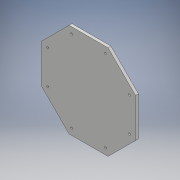
# Autodesk Inventor part: meteostanica radiation shield spodny kryt
Saved by Autodesk Inventor 2017 (Build 210142000, 142)
## iProperties
Created: 2017-02-23
Part Number: meteostanica radiation shield spodny kryt
Material: Generic
Document SubType Name: Modeling
Designer: Luc3as
Density: 1 g/cm^3
Appearance: Default
Author: Luc3as
Autodesk Inventor part; units mm, degrees
ref_plane "YZ Plane" through (0, 0, 0) normal (1, 0, 0) x (0, 1, 0)
ref_plane "XZ Plane" through (0, 0, 0) normal (0, 1, 0) x (-1, 0, 0)
ref_plane "XY Plane" through (0, 0, 0) normal (0, 0, 1) x (1, 0, 0)
ref_plane "Work Plane13" through (0, 0, 0) normal (0, -1, 0) x (1, 0, 0)
sketch "Sketch13" plane through (0, 0, 0) normal (0, -1, 0) x (1, 0, 0)
  circle A0 centre (-71.6992, -29.6988) radius 0.75 projected
  circle A1 centre (29.6988, -71.6992) radius 0.75 projected
  circle A2 centre (71.6992, 29.6988) radius 0.75 projected
  circle A3 centre (29.6988, 71.6992) radius 0.75 projected
  circle A4 centre (-29.6988, 71.6992) radius 0.75 projected
  circle A5 centre (71.6992, -29.6988) radius 0.75 projected
  circle A6 centre (-29.6988, -71.6992) radius 0.75 projected
  circle A7 centre (-71.6992, 29.6988) radius 0.75 projected
  line L0 (-82.6875, -34.2503) -> (-34.2503, -82.6875) projected
  line L1 (-34.2503, -82.6875) -> (34.2503, -82.6875) projected
  line L2 (34.2503, -82.6875) -> (82.6875, -34.2503) projected
  line L3 (82.6875, -34.2503) -> (82.6875, 34.2503) projected
  line L4 (82.6875, 34.2503) -> (34.2503, 82.6875) projected
  line L5 (34.2503, 82.6875) -> (-34.2503, 82.6875) projected
  line L6 (-34.2503, 82.6875) -> (-82.6875, 34.2503) projected
  line L7 (-82.6875, 34.2503) -> (-82.6875, -34.2503) projected
  arc A8 (-33.3536, 70.0737) -> (-25.965, 73.1342) centre (-29.6988, 71.6992) ccw projected
  arc A9 (25.965, 73.1342) -> (-25.965, 73.1342) centre (0, 0) ccw projected
  arc A10 (25.965, 73.1342) -> (33.3536, 70.0737) centre (29.6988, 71.6992) ccw projected
  arc A11 (70.0737, 33.3536) -> (33.3536, 70.0737) centre (0, 0) ccw projected
  arc A12 (70.0737, 33.3536) -> (73.1342, 25.965) centre (71.6992, 29.6988) ccw projected
  arc A13 (73.1342, -25.965) -> (73.1342, 25.965) centre (0, 0) ccw projected
  arc A14 (73.1342, -25.965) -> (70.0737, -33.3536) centre (71.6992, -29.6988) ccw projected
  arc A15 (33.3536, -70.0737) -> (70.0737, -33.3536) centre (0, 0) ccw projected
  arc A16 (33.3536, -70.0737) -> (25.965, -73.1342) centre (29.6988, -71.6992) ccw projected
  arc A17 (-25.965, -73.1342) -> (25.965, -73.1342) centre (0, 0) ccw projected
  arc A18 (-25.965, -73.1342) -> (-33.3536, -70.0737) centre (-29.6988, -71.6992) ccw projected
  arc A19 (-70.0737, -33.3536) -> (-33.3536, -70.0737) centre (0, 0) ccw projected
  arc A20 (-70.0737, -33.3536) -> (-73.1342, -25.965) centre (-71.6992, -29.6988) ccw projected
  arc A21 (-73.1342, 25.965) -> (-73.1342, -25.965) centre (0, 0) ccw projected
  arc A22 (-73.1342, 25.965) -> (-70.0737, 33.3536) centre (-71.6992, 29.6988) ccw projected
  arc A23 (-33.3536, 70.0737) -> (-70.0737, 33.3536) centre (0, 0) ccw projected
extrude "Extrusion11" add sketch "Sketch13" along normal blind 5 contours L7 L6 L5 L4 L3 L2 L1 L0 | A8 A9 A10 A11 A12 A13 A14 A15 A16 A17 A18 A19 A20 A21 A22 A23
chamfer "Chamfer2" distance 1 angle 45 8 edges at (-72.4492, -5, -29.6988) (-30.4488, -5, -71.6992) (28.9488, -5, -71.6992) (70.9492, -5, -29.6988) (70.9492, -5, 29.6988) (28.9488, -5, 71.6992) (-30.4488, -5, 71.6992) (-72.4492, -5, 29.6988)
body "Solid1"
